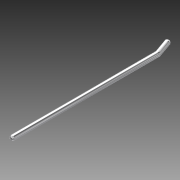
# Autodesk Inventor part: LandingSkid
Saved by Autodesk Inventor 2011 SP1 (Build 150282100, 282)
## iProperties
Created: 2011-08-02
Part Number: LandingSkid
Document SubType Name: Modeling
Designer: Nathan
Density: 1 g/cm^3
Author: Nathan
Autodesk Inventor part; units mm, degrees
ref_plane "YZ Plane" through (0, 0, 0) normal (1, 0, 0) x (0, 1, 0)
ref_plane "XZ Plane" through (0, 0, 0) normal (0, 1, 0) x (-1, 0, 0)
ref_plane "XY Plane" through (0, 0, 0) normal (0, 0, 1) x (1, 0, 0)
sketch "Sketch1" plane through (0, 0, 0) normal (0, 0, 1) x (1, 0, 0)
  circle A0 centre (0, 0) radius 4.7625
  dimension "d0" = 9.525
  constraints: 1 centre point, 1 coincident
  measures "d0" diameter of A0
sketch "Sketch3" plane through (0, 0, 0) normal (1, 0, 0) x (0, 1, 0)
  line L0 (4.7625, 0) -> (-4.7625, 0) projected
  line L1 (0, 0) -> (0, -292.1)
  line L2 (0, -292.1) -> (12.19, -314.3837)
  dimension "d1" = 292.1
  dimension "d2" = 25.4
  constraints: 4 end point, 1 perpendicular
  measures "d1" distance of L1.start L1.end
  measures "d2" distance of L1.end L2.end
sweep "Sweep1" add profiles "Sketch1" path "Sketch3" path curves L1 L2
fillet "Fillet1" radius 9.525 1 edges at (0, 4.7625, -290.8825)
fillet "Fillet2" radius 2.54 2 edges at (3.3676, -3.3676, -292.9609) (-3.3676, -3.3676, -292.9609)
fillet "Fillet3" radius 4.1275 1 edges at (-4.7625, 0, 0)
fillet "Fillet4" radius 4.1275 1 edges at (-4.7625, 12.19, -314.3837)
body "Solid1"
